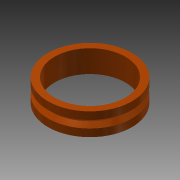
# Autodesk Inventor part: z idler
Saved by Autodesk Inventor 2014 (Build 180170000, 170)
## iProperties
Created: 2013-10-16
Part Number: z idler
Material: Generic
Document SubType Name: Modeling
Designer: employee
Density: 1 g/cm^3
Mass: 0.993604 g
Surface Area: 14.5028 cm^2
Volume: 0.993604 cm^3
Appearance: Smooth - Light Orange
Author: employee
Autodesk Inventor part; units mm, degrees
ref_plane "YZ Plane" through (0, 0, 0) normal (1, 0, 0) x (0, 1, 0)
ref_plane "XZ Plane" through (0, 0, 0) normal (0, 1, 0) x (-1, 0, 0)
ref_plane "XY Plane" through (0, 0, 0) normal (0, 0, 1) x (1, 0, 0)
sketch "Sketch1" plane through (0, 0, 0) normal (0, 1, 0) x (-1, 0, 0)
  line L0 (11.1, 0) -> (11.1, 7)
  line L1 (11.1, 7) -> (13.1667, 7)
  line L2 (13.1667, 7) -> (13.1667, 4.6667)
  line L3 (13.1667, 4.6667) -> (12, 3.5)
  line L4 (12, 3.5) -> (13.1667, 2.3333)
  line L5 (13.1667, 2.3333) -> (13.1667, 0)
  line L6 (13.1667, 0) -> (11.1, 0)
  line L7 (0, 0) -> (0, 4.5986)
  line L8 (13.1667, 4.6667) -> (13.1667, 2.3333)
  dimension "d0" = 11.1
  dimension "d3" = 7
  dimension "d4" = 12
  constraints: 18 end point, 4 equal length, 4 parallel, 3 perpendicular, 1 horizontal alignment, 1 vertical
  measures "d0" distance between parallel lines of L0 L7
  measures "d3" distance of L0.start L0.end
  measures "d4" distance from line of L3.end L7
revolve "Revolution1" add sketch "Sketch1" angle 360 about axis through (0, 0, 0) along (0, 0, 1) contours L0 L1 L2 L3 L4 L5 L6
body "Solid1"
